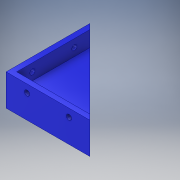
# Autodesk Inventor part: bracket
Saved by Autodesk Inventor 2017 (Build 210142000, 142)
## iProperties
Created: 2019-02-16
Part Number: bracket
Material: Generic
Document SubType Name: Modeling
Designer: Mitch
Density: 1 g/cm^3
Appearance: Blue - Wall Paint - Glossy
Author: Mitch
Autodesk Inventor part; units mm, degrees
ref_plane "YZ Plane" through (0, 0, 0) normal (1, 0, 0) x (0, 1, 0)
ref_plane "XZ Plane" through (0, 0, 0) normal (0, 1, 0) x (-1, 0, 0)
ref_plane "XY Plane" through (0, 0, 0) normal (0, 0, 1) x (1, 0, 0)
sketch "Sketch1" plane through (0, 0, 0) normal (0, 1, 0) x (-1, 0, 0)
  line L0 (0, 0) -> (101.6, 0)
  line L1 (101.6, 0) -> (101.6, -101.6)
  line L2 (0, 0) -> (101.6, -101.6)
  dimension "d2" = 101.6
  dimension "d3" = 101.6
  constraints: 6 end point, 1 horizontal, 1 perpendicular
  measures "d2" distance of L0.end L1.end
  measures "d3" distance of L0.start L0.end
extrude "Extrusion1" add sketch "Sketch1" along normal blind 38.1
sketch "Sketch2" plane through (0, 38.1, 0) normal (0, 1, 0) x (1, 0, 0)
  line L0 (-101.6, 0) -> (0, 0) projected
  line L1 (-101.6, 101.6) -> (-101.6, 0) projected
  line L2 (-6.35, 6.35) -> (-95.25, 6.35)
  line L3 (-95.25, 6.35) -> (-95.25, 95.25)
  line L4 (0, 0) -> (-101.6, 101.6) projected
  line L5 (-6.35, 6.35) -> (-95.25, 95.25)
  dimension "d6" = 6.35
  constraints: 6 end point, 2 point on line
  measures "d6" distance between parallel lines of L0 L2
extrude "Extrusion2" cut sketch "Sketch2" against normal blind 19.05 contours L2 L3 L4
hole "Hole1" at (-95.25, 28.575, -76.2) direction (-1, 0, 0) diameter 6.35 end through all
hole "Hole2" at (-95.25, 28.575, -25.4) direction (-1, 0, 0) diameter 6.35 end through all
hole "Hole3" at (-25.4, 28.575, -6.35) direction (0, 0, 1) diameter 6.35 end through all
hole "Hole4" at (-76.2, 28.575, -6.35) direction (0, 0, 1) diameter 6.35 end through all
sketch "Sketch3" plane through (0, 0, 0) normal (0, -1, 0) x (1, 0, 0)
  line L0 (-74.5236, -579.4502) -> (246.1514, -579.4502) projected
  line L1 (-74.5236, -34.9377) -> (-74.5236, -579.4502) projected
  line L2 (246.1514, -34.9377) -> (-74.5236, -34.9377) projected
  line L3 (246.1514, -579.4502) -> (246.1514, -34.9377) projected
  line L4 (-74.5236, -34.9377) -> (-74.5236, -74.5236)
  line L5 (-101.6, -101.6) -> (0, 0) projected
  line L6 (-34.8701, -34.9377) -> (-74.5236, -34.9377)
  line L7 (-34.8701, -34.9377) -> (-74.5236, -74.5236)
  constraints: 6 end point, 3 point on line, 1 perpendicular
extrude "Extrusion3" cut sketch "Sketch3" against normal blind 9.7282 contours L1 L2 L5 | L5 L2 L7
body "Solid1"
